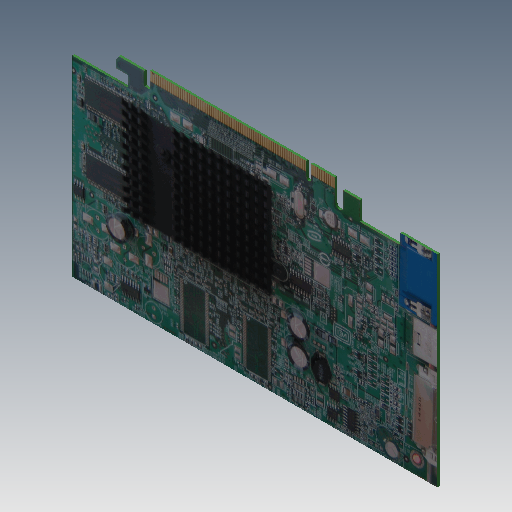
# Autodesk Inventor part: config - graphic card
Saved by Autodesk Inventor 2019.1 (Build 231200000, 200)
## iProperties
Company: Autodesk Asia Pte. Ltd.
Created: 2005-12-11
Part Number: config - graphic card
Document SubType Name: Modeling
Designer: Simon.Ng@autodesk.com
Stock Number: config - graphic card
Density: 1 g/cm^3
Material: Generic
Mass: 16.0813 g
Surface Area: 327.607 cm^2
Volume: 16.0813 cm^3
Appearance: Smooth - Dark Forest Green
Title: PC Demo
Author: Simon.Ng@autodesk.com
Autodesk Inventor part; units mm, degrees
ref_plane "YZ Plane" through (0, 0, 0) normal (1, 0, 0) x (0, 1, 0)
ref_plane "XZ Plane" through (0, 0, 0) normal (0, 1, 0) x (-1, 0, 0)
ref_plane "XY Plane" through (0, 0, 0) normal (0, 0, 1) x (1, 0, 0)
sketch "Sketch1" plane through (0, 0, 0) normal (0, 0, 1) x (1, 0, 0)
  line L0 (0, 96) -> (0, -72) projected
  line L1 (-18, 0) -> (234, 0) projected
  line L2 (0, 60) -> (180, 60)
  line L3 (180, 60) -> (180, -60)
  line L4 (180, -60) -> (0, -60)
  line L5 (0, -60) -> (0, 60)
  dimension "d0" = 180
  dimension "d1" = 120
  constraints: 8 end point, 2 parallel, 1 horizontal, 1 perpendicular, 1 point on line, 1 other
  measures "d0" distance of L3.end L4.end
  measures "d1" distance of L2.end L3.end
extrude "Extrusion1" add sketch "Sketch1" along normal blind 1
decal "Decal2"
decal "Decal3"
sketch "Sketch5" plane through (0, 0, 1) normal (0, 0, 1) x (1, 0, 0)
  line L0 (0, 60) -> (180, 60) projected
  line L1 (0, -60) -> (0, 60) projected
  line L2 (180, -60) -> (0, -60) projected
  line L3 (0, 38.2522) -> (25.6905, 38.2522)
  line L4 (25.6905, 38.2522) -> (25.6905, 43.1713)
  line L5 (25.6905, 43.1713) -> (19.893, 43.1713)
  line L6 (19.893, 43.1713) -> (19.893, 46.2458)
  line L7 (19.893, 46.2458) -> (21.3863, 48.6175)
  line L8 (21.3863, 48.6175) -> (33.1461, 48.6175)
  line L9 (33.1461, 48.6175) -> (33.1461, 42.5564)
  line L10 (33.1461, 42.5564) -> (35.7923, 42.5564)
  line L11 (35.7923, 42.5564) -> (35.7923, 60)
  line L12 (120.7923, 60) -> (124.7021, 60)
  line L13 (124.7021, 60) -> (124.7021, 40.0365)
  line L14 (124.7021, 40.0365) -> (120.7923, 40.0365)
  line L15 (120.7923, 40.0365) -> (120.7923, 60)
  circle A0 centre (122.7472, 40.0365) radius 1.9549
  line L16 (35.7923, 50.0951) -> (120.7923, 50.0183)
  line L17 (107.7365, 50.0301) -> (109.8537, 50.0301)
  line L18 (109.8537, 50.0301) -> (109.8537, 43.66)
  line L19 (109.8537, 43.66) -> (107.7365, 43.66)
  line L20 (107.7365, 43.66) -> (107.7365, 50.0301)
  circle A1 centre (108.7951, 43.66) radius 1.0586
  dimension "d14" = 85
  constraints: 36 end point, 10 parallel, 5 point on line, 4 perpendicular, 3 midpoint, 2 horizontal, 2 horizontal alignment, 4 other
  measures "d14" distance between parallel lines of L15 L11
extrude "Extrusion2" cut sketch "Sketch5" against normal through all
sketch "Sketch6" plane through (0, 0, 1) normal (0, 0, 1) x (1, 0, 0)
  line L0 (124.7021, 60) -> (124.7021, 40.0365) projected
  line L1 (0, -60) -> (0, 38.2522) projected
  line L2 (180, -60) -> (0, -60) projected
  line L3 (180, 60) -> (180, -60) projected
  line L4 (124.7021, 60) -> (180, 60) projected
  line L5 (124.7021, 46.8108) -> (132.4781, 46.8108)
  line L6 (132.4781, 46.8108) -> (132.4781, 38.2477)
  line L7 (168, -50) -> (0, -50)
  line L8 (-18, 0) -> (234, 0) projected
  line L9 (168, 43) -> (168, -50)
  line L10 (132.4781, 38.2477) -> (150.9588, 38.2477)
  line L11 (150.9588, 38.2477) -> (150.9588, 43)
  line L12 (150.9588, 43) -> (168, 43)
  dimension "d16" = 93
  dimension "d17" = 10
  dimension "d18" = 168
  constraints: 14 end point, 4 perpendicular, 3 parallel, 2 point on line
  measures "d16" distance of L9.start L7.start
  measures "d17" distance between parallel lines of L2 L7
  measures "d18" distance between parallel lines of L1 L9
extrude "Extrusion3" cut sketch "Sketch6" against normal through all contours L4 L3 L8 L9 L12 L11 L10 L6 L5 L0 | L3 L2 L1 L7 L9 L8
sketch "Sketch3" plane through (0, 0, 1) normal (0, 0, 1) x (1, 0, 0)
  line L0 (0, 50.1511) -> (168, 50.1511) construction
  line L1 (168, 50.1511) -> (168, -50.153) construction
  line L2 (168, -50.153) -> (0, -50.153) construction
  line L3 (0, -50.153) -> (0, 50.1511) construction
  point P0 (0, 0)
  point P1 (0, 0)
  constraints: 2 coincident, 4 other
sketch "Sketch4" plane through (0, 0, 0) normal (0, 0, -1) x (-1, 0, 0)
  line L0 (0, -60) -> (0, 60) projected
  line L1 (-165.5, 50.5194) -> (0, 50.5194) construction
  line L2 (0, 50.5194) -> (0, -50.5196) construction
  line L3 (0, -50.5196) -> (-165.5, -50.5196) construction
  line L4 (-165.5, -50.5196) -> (-165.5, 50.5194) construction
  point P0 (0, 0)
  point P1 (0, 0)
  point P2 (0, -50.5196)
  constraints: 2 coincident, 1 midpoint, 4 other
body "Solid1"
